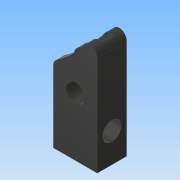
# Autodesk Inventor part: standLegs
Saved by Autodesk Inventor 2017.3 (Build 213256000, 256)
## iProperties
Created: 2019-05-30
Part Number: standLegs
Material: Acetal Resin, Black
Document SubType Name: Modeling
Designer: Derek Wider
Density: 1.425 g/cm^3
Appearance: Smooth - Black
Author: Derek Wider
Autodesk Inventor part; units mm, degrees
ref_plane "YZ Plane" through (0, 0, 0) normal (1, 0, 0) x (0, 1, 0)
ref_plane "XZ Plane" through (0, 0, 0) normal (0, 1, 0) x (-1, 0, 0)
sketch "Sketch1" plane through (0, 0, 0) normal (0, 0, 1) x (1, 0, 0)
  line L0 (0, 0) -> (19.05, 0)
  line L1 (19.05, 0) -> (19.05, 57.15)
  line L2 (19.05, 57.15) -> (0, 57.15)
  line L3 (0, 57.15) -> (0, 0)
  circle A0 centre (9.525, 25.4) radius 4.064
  circle A1 centre (-25.4, 73.025) radius 47.625
  point P0 (9.525, 57.15)
  dimension "d0" = 19.05
  dimension "d1" = 57.15
  dimension "d2" = 8.128
  dimension "d3" = 25.4
  dimension "d6" = 95.25
  dimension "d7" = 25.4
  dimension "d8" = 73.025
  constraints: 8 end point, 2 centre point, 2 parallel, 1 horizontal, 1 midpoint, 1 perpendicular, 1 vertical alignment
  measures "d0" distance of L2.end L1.end
  measures "d1" distance of L1.end L0.end
  measures "d2" diameter of A0
  measures "d3" distance from line of L0 A0.centre
  measures "d6" diameter of A1
  measures "d7" horizontal distance of L0.start A1.centre
  measures "d8" vertical distance of L0.start A1.centre
extrude "Extrusion1" add sketch "Sketch1" along normal blind 12.7 contours L3 A1 L1 L0 | L3 L2 L1 A1 picked at (2.0344, 42.399)
extrude "Extrusion2" cut sketch "Sketch1" along normal blind 12.7 contours A1 L1 L2 L3 | L3 L2 L1 A1
sketch "Sketch2" plane through (19.05, 0, 0) normal (1, 0, 0) x (0, 0, -1)
  circle A0 centre (-6.35, 12.7) radius 4.064
  line L0 (0, 0) -> (0, 55.9271) construction
  line L1 (-12.7, 0) -> (-12.7, 55.9271) construction
  line L2 (0, 0) -> (-12.7, 0) construction
  line L3 (0, 55.9271) -> (-12.7, 55.9271) projected
  point P0 (0, 0)
  point P1 (-6.35, 47.625)
  dimension "d13" = 8.128
  dimension "d16" = 12.7
  constraints: 1 centre point, 1 vertical alignment
  measures "d13" diameter of A0
  measures "d16" distance from line of L2 A0.centre
extrude "Extrusion3" cut sketch "Sketch2" against normal through all
ref_plane "Work Plane1" through (0, 0, 6.35) normal (0, 0, 1) x (1, 0, 0)
sketch "Sketch3" plane through (0, 0, 6.35) normal (0, 0, 1) x (1, 0, 0)
  arc A0 (0, 32.7388) -> (19.05, 55.9271) centre (-25.4, 73.025) ccw construction
  circle A1 centre (-25.4, 73.025) radius 49.53
  point P0 (0, 0)
  dimension "d18" = 99.06
  constraints: 1 centre point, 1 coincident
  measures "d18" diameter of A1
extrude "Extrusion4" cut sketch "Sketch3" along normal mid plane 3.175
fillet "Fillet1" radius 3.175 4 edges at (19.05, 55.9271, 2.3812) (0, 32.7388, 10.3187) (0, 30.5037, 6.35) (0, 32.7388, 2.3812)
fillet "Fillet2" radius 1.27 10 edges at (14.6879, 46.3553, 4.7625) (0.3687, 32.5087, 4.7625) (0, 30.7637, 4.7625) (0, 29.6211, 4.7625) (7.853, 38.9314, 4.7625) (0.3687, 32.5087, 7.9375) (0, 30.7637, 7.9375) (0, 29.6211, 7.9375) (14.6879, 46.3553, 7.9375) (7.853, 38.9314, 7.9375)
fillet "Fillet3" radius 1.27 1 edges at (16.4497, 46.5331, 6.35)
body "Solid1"
